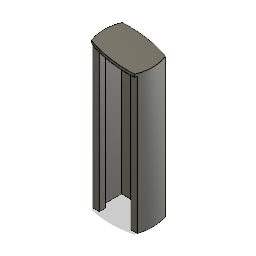
Sensor Cover Left v1 (Autodesk Fusion 360 design; units mm, degrees)
Autodesk Fusion 360 part; units mm, degrees
sketch "Sketch1" plane through (0, 0, 0) normal (0, 1, 0) x (1, 0, 0)
  line L0 (25, 18) -> (-25, 18) construction
  line L1 (-25, 18) -> (-25, -18) construction
  line L2 (-25, -18) -> (25, -18) construction
  line L3 (25, -18) -> (25, 18) construction
  line L4 (25, 18) -> (-25, -18) construction
  line L5 (-25, 18) -> (25, -18) construction
  arc A0 (25, 18) -> (-25, 18) centre (0, -84.6667) ccw
  arc A1 (-25, -18) -> (25, -18) centre (0, 84.6667) ccw
  arc A2 (25, -18) -> (25, 18) centre (-27.5, 0) ccw
  arc A3 (-25, 18) -> (-25, -18) centre (27.5, 0) ccw
  arc A4 (-23.0621, -15.8893) -> (23.0621, -15.8893) centre (0, 84.6667) ccw
  arc A5 (23.0621, -15.8893) -> (23.0621, 15.8893) centre (-27.5, 0) ccw
  arc A6 (23.0621, 15.8893) -> (-23.0621, 15.8893) centre (0, -84.6667) ccw
  arc A7 (-23.0621, 15.8893) -> (-23.0621, -15.8893) centre (27.5, 0) ccw
  dimension "d1" = 50
  dimension "d2" = 36
  dimension "d3" = 42
  dimension "d4" = 56
  dimension "d5" = 2.5
extrude "Extrude1" add sketch "Sketch1" along normal blind 170
sketch "Sketch3" plane through (0, 0, 0) normal (0, -1, 0) x (-1, 0, 0)
  arc A0 (23.0621, -15.8893) -> (23.0621, 15.8893) centre (-27.5, 0) ccw
  arc A1 (-23.0621, -15.8893) -> (23.0621, -15.8893) centre (0, 84.6667) ccw
  arc A2 (-23.0621, 15.8893) -> (-23.0621, -15.8893) centre (27.5, 0) ccw
  arc A3 (23.0621, 15.8893) -> (-23.0621, 15.8893) centre (0, -84.6667) ccw
  arc A4 (25, -18) -> (25, 18) centre (-27.5, 0) ccw
  arc A5 (25, 18) -> (-25, 18) centre (0, -84.6667) ccw
  arc A6 (-25, 18) -> (-25, -18) centre (27.5, 0) ccw
  arc A7 (-25, -18) -> (25, -18) centre (0, 84.6667) ccw
  line L0 (-23, -1) -> (23, -1)
  line L1 (23, -1) -> (23, 15)
  line L2 (23, 15) -> (-23, 15)
  line L3 (-23, 15) -> (-23, -1)
  line L4 (-23, -1) -> (23, 15) construction
  line L5 (23, -1) -> (-23, 15) construction
  arc A8 (23.0621, -15.8893) -> (23.0621, 15.8893) centre (-27.5, 0) ccw
  arc A9 (-23.0621, -15.8893) -> (23.0621, -15.8893) centre (0, 84.6667) ccw
  arc A10 (-23.0621, 15.8893) -> (-23.0621, -15.8893) centre (27.5, 0) ccw
  arc A11 (23.0621, 15.8893) -> (-23.0621, 15.8893) centre (0, -84.6667) ccw
  arc A12 (25, -18) -> (25, 18) centre (-27.5, 0) ccw
  arc A13 (25, 18) -> (-25, 18) centre (0, -84.6667) ccw
  arc A14 (-25, 18) -> (-25, -18) centre (27.5, 0) ccw
  arc A15 (-25, -18) -> (25, -18) centre (0, 84.6667) ccw
  arc A16 (23.0621, -15.8893) -> (23.0621, 15.8893) centre (-27.5, 0) ccw
  arc A17 (23.0621, 15.8893) -> (-23.0621, 15.8893) centre (0, -84.6667) ccw
  arc A18 (-23.0621, 15.8893) -> (-23.0621, -15.8893) centre (27.5, 0) ccw
  arc A19 (-23.0621, -15.8893) -> (23.0621, -15.8893) centre (0, 84.6667) ccw
  arc A20 (25, -18) -> (25, 18) centre (-27.5, 0) ccw
  arc A21 (-25, -18) -> (25, -18) centre (0, 84.6667) ccw
  arc A22 (-25, 18) -> (-25, -18) centre (27.5, 0) ccw
  arc A23 (25, 18) -> (-25, 18) centre (0, -84.6667) ccw
  line L6 (23, -1) -> (23, -8.5)
  line L7 (23, -8.5) -> (18, -8.5)
  line L8 (18, -8.5) -> (18, -16.9176)
  line L9 (-23, -1) -> (-23, -8.5)
  line L10 (-23, -8.5) -> (-18, -8.5)
  line L11 (-18, -8.5) -> (-18, -16.9176)
  dimension "d10" = 16
  dimension "d11" = 46
  dimension "d12" = 6
  dimension "d33" = 23.5
  dimension "d34" = 36
  measures "d10" distance of origin
  measures "d12" distance of L2
  measures "d33" distance of L2 L10
  measures "d34" distance of L8 L11
extrude "Extrude3" add sketch "Sketch3" against normal blind 170 contours A0 A1 A2 A3 L1 L2 L3 A8 A9 A10 A11 A16 A17 A18 A19 L6 L7 L8 L9 L10 L11
ref_plane "WorkPlane4" through (0, 150, 0) normal (0, 1, 0) x (0, 0, 1)
sketch "Sketch11" plane through (0, 150, 0) normal (0, 1, 0) x (1, 0, 0)
  line L0 (-18, -16.9176) -> (-18, -8.5)
  line L1 (-18, -8.5) -> (-23, -8.5)
  line L2 (-23, -8.5) -> (-23, 15)
  line L3 (-23, 15) -> (23, 15)
  line L4 (23, 15) -> (23, -8.5)
  line L5 (23, -8.5) -> (18, -8.5)
  line L6 (18, -8.5) -> (18, -16.9176)
  arc A0 (-18, -16.9176) -> (18, -16.9176) centre (0, 84.6667) ccw
  arc A1 (-25, 18) -> (-25, -18) centre (27.5, 0) ccw
  arc A2 (-25, -18) -> (25, -18) centre (0, 84.6667) ccw
  arc A3 (25, -18) -> (25, 18) centre (-27.5, 0) ccw
  arc A4 (25, 18) -> (-25, 18) centre (0, -84.6667) ccw
extrude "Extrude8" add sketch "Sketch11" along normal up to surface (20 mm away) contours L0 L1 L2 L3 L4 L5 L6 A0
sketch "Sketch8" plane through (0, 0, 0) normal (0, 0, 1) x (1, 0, 0)
  line L0 (-28, 170) -> (28, 160)
  line L1 (25, 0) -> (25, 170)
  line L2 (28, 160) -> (28, 210.2672)
  line L3 (28, 210.2672) -> (-28, 210.2672)
  line L4 (-28, 210.2672) -> (-28, 170)
  line L5 (28, 0) -> (25, 0)
  line L6 (-25, 0) -> (-28, 0)
  dimension "d35" = 160
  dimension "d36" = 170
extrude "Extrude7" cut sketch "Sketch8" along normal through all and the other way through all
ref_plane "WorkPlane3" through (-0.5274, 162.0467, 0) normal (0.175791, 0.984428, 0) x (-0.984428, 0.175791, 0)
sketch "Sketch12" plane through (0, 0, 0) normal (0, -1, 0) x (1, 0, 0)
  arc A0 (18, 16.9176) -> (-18, 16.9176) centre (0, -84.6667) ccw
  line L0 (18, 16.9176) -> (18, 8.5)
  line L1 (18, 8.5) -> (23, 8.5)
  line L2 (23, 8.5) -> (23, -15)
  line L3 (23, -15) -> (-23, -15)
  line L4 (-23, -15) -> (-23, 8.5)
  line L5 (-23, 8.5) -> (-18, 8.5)
  line L6 (-18, 8.5) -> (-18, 16.9176)
  arc A1 (-25, 18) -> (-25, -18) centre (27.5, 0) ccw
  arc A2 (-25, -18) -> (25, -18) centre (0, 84.6667) ccw
  arc A3 (25, -18) -> (25, 18) centre (-27.5, 0) ccw
  arc A4 (25, 18) -> (-25, 18) centre (0, -84.6667) ccw
extrude "Extrude9" cut sketch "Sketch12" along normal up to surface contours A0 L0 L1 L2 L3 L4 L5 L6 end surface through (-0.5274, 162.0467, 0) normal (0.175791, 0.984428, 0) offset 0
sketch "Sketch9" plane through (0, 0, 0) normal (0, -1, 0) x (1, 0, 0)
  arc A0 (18, 16.9176) -> (-18, 16.9176) centre (0, -84.6667) ccw
  line L0 (18, 16.9176) -> (18, 8.5)
  line L1 (18, 8.5) -> (23, 8.5)
  line L2 (23, 8.5) -> (23, -15)
  line L3 (23, -15) -> (-23, -15)
  line L4 (-23, -15) -> (-23, 8.5)
  line L5 (-23, 8.5) -> (-18, 8.5)
  line L6 (-18, 8.5) -> (-18, 16.9176)
  arc A1 (-25, 18) -> (-25, -18) centre (27.5, 0) ccw
  arc A2 (-25, -18) -> (25, -18) centre (0, 84.6667) ccw
  arc A3 (25, -18) -> (25, 18) centre (-27.5, 0) ccw
  arc A4 (25, 18) -> (-25, 18) centre (0, -84.6667) ccw
  line L7 (-33, 32.4232) -> (28, 32.4232)
  line L8 (28, 32.4232) -> (28, 15.5)
  line L9 (28, 15.5) -> (-33, 15.5)
  line L10 (-33, 15.5) -> (-33, 32.4232)
  dimension "d39" = 7
  measures "d39" distance of L5 L9
extrude "Extrude10" cut sketch "Sketch9" along normal up to surface contours A0 L0 L6 A1 A3 A4 L9 end surface through (-0.5274, 162.0467, 0) normal (0.175791, 0.984428, 0) offset 0
